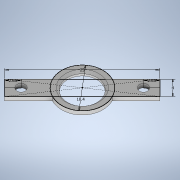
# Autodesk Inventor part: Headplate_2p
Saved by Autodesk Inventor 2022 (Build 260153000, 153)
## iProperties
Created: 2022-06-15
Part Number: Headplate_2p
Material: Generic
Document SubType Name: Modeling
Designer: Sylvia
Density: 1 g/cm^3
Appearance: Default
Author: Sylvia
Autodesk Inventor part; units mm, degrees
ref_plane "YZ Plane" through (0, 0, 0) normal (1, 0, 0) x (0, 1, 0)
ref_plane "XZ Plane" through (0, 0, 0) normal (0, 1, 0) x (-1, 0, 0)
ref_plane "XY Plane" through (0, 0, 0) normal (0, 0, 1) x (1, 0, 0)
sketch "Sketch1" plane through (0, 0, 0) normal (0, 1, 0) x (-1, 0, 0)
  circle A0 centre (0, 0) radius 5.2
  line L0 (2, 12.5) -> (-2, 12.5)
  line L1 (-2, 12.5) -> (-2, -12.5)
  line L2 (-2, -12.5) -> (2, -12.5)
  line L3 (2, -12.5) -> (2, 12.5)
  line L4 (2, 12.5) -> (-2, -12.5) construction
  line L5 (-2, 12.5) -> (2, -12.5) construction
  line L6 (0, 12.5) -> (0, 9.85)
  line L7 (0, -12.5) -> (0, -9.85)
  point P0 (-2, 4.8)
  point P1 (-2, -4.8)
  point P2 (2, -4.8)
  point P3 (2, 4.8)
  dimension "d0" = 10.4
  dimension "d1" = 4
  dimension "d2" = 25
  dimension "d19" = 2.65
  dimension "d20" = 2.65
  constraints: 16 end point, 4 midpoint, 2 parallel, 2 vertical, 1 centre point, 1 coincident, 1 horizontal, 1 perpendicular
  measures "d0" diameter of A0
  measures "d1" distance of L2.end L1.end
  measures "d2" distance of L1.end L0.end
  measures "d19" distance of L6.start L6.end
  measures "d20" distance of L7.start L7.end
extrude "Extrusion1" add sketch "Sketch1" along normal blind 1
hole "Hole2" at (0, 0, 0) direction (0, 1, 0) diameter 7.4 depth 1 tip angle 118 countersink diameter 8.4 countersink angle 90
hole "Hole3" at (0, 0, 9.85) direction (0, 1, 0) diameter 2 depth 1 tip angle 118
hole "Hole4" at (0, 0, -9.85) direction (0, 1, 0) diameter 2 depth 1 tip angle 118
body "Solid1"
